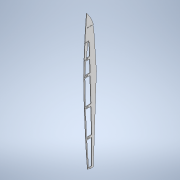
# Autodesk Inventor part: stinger
Saved by Autodesk Inventor 2020.3 (Build 243373010, 373A)
## iProperties
Created: 2020-05-20
Part Number: stinger
Material: Generic
Document SubType Name: Modeling
Designer: kardo
Density: 1 g/cm^3
Appearance: Default
Mass: 15.45 g
Surface Area: 197.993 cm^2
Volume: 15.45 cm^3
Author: kardo
Autodesk Inventor part; units mm, degrees
ref_plane "YZ Plane" through (0, 0, 0) normal (1, 0, 0) x (0, 1, 0)
ref_plane "XZ Plane" through (0, 0, 0) normal (0, 1, 0) x (-1, 0, 0)
ref_plane "XY Plane" through (0, 0, 0) normal (0, 0, 1) x (1, 0, 0)
derived "base_sketch.ipt"
sketch "stringer" plane through (0, 0, 0) normal (1, 0, 0) x (0, 1, 0)
  line L0 (-306, 11.475) -> (0, 0)
  line L1 (-306, 31.875) -> (-306, 11.475)
  line L2 (-412.4622, 0) -> (310.4457, 0)
  line L3 (0, -13.6228) -> (0, 64.3297)
  line L4 (0, 0) -> (122.4, 8.559)
  line L5 (-306, 31.875) -> (-153, 45.9) construction
  line L6 (-153, 45.9) -> (0, 45.9) construction
  line L7 (0, 45.9) -> (102, 45.9) construction
  line L8 (102, 45.9) -> (204, 35.7) construction
  line L9 (122.4, 8.559) -> (204, 14.2651) construction
  spline S0 degree 4 poles (-306, 31.875) (-229.6805, 38.871) (-153.0004, 41.6957) (-76.5755, 45.9) (0, 45.9) knots 0 0 0 0 0 1 1 1 1 1
  spline S1 degree 4 poles (0, 45.9) (51.0599, 45.9) (102.0004, 42.8427) (153.143, 40.7857) (204, 35.7) knots 0 0 0 0 0 1 1 1 1 1
  spline S2 degree 4 poles (122.4, 8.559) (129.6243, 9.0642) (155.3021, 10.8598) (183.5774, 20.1745) (192.0601, 27.4338) (204, 35.7) knots 0 0 0 0 0 0.281346 1 1 1 1 1
  point P0 (-153, 41.6925)
  point P1 (102, 42.84)
  point P2 (163.2, 15.056)
  point P3 (187.68, 24.9131)
sketch "bulkhead_main" plane through (0, 0, 0) normal (0, 1, 0) x (-1, 0, 0)
  line L0 (0, 19.935) -> (28.764, 19.935)
  line L1 (28.764, 19.935) -> (28.764, 13.529)
  line L2 (28.764, 13.529) -> (62.322, 13.529)
  line L3 (0, 0) -> (-11.5056, 0)
  line L4 (-11.5056, 0) -> (-11.5056, -2.4868)
  line L5 (-11.5056, -2.4868) -> (-34.5168, -2.4868)
  line L6 (-34.5168, -2.4868) -> (-57.528, 27.54)
  line L7 (19.176, 46.818) -> (62.322, 46.818)
  line L8 (0, 19.935) -> (0, 0)
  line L9 (86.7165, 0) -> (-84.045, 0)
  line L10 (0, -13.6228) -> (0, 64.3297)
  line L11 (62.322, 46.818) -> (62.322, 13.529)
  spline S0 degree 4 poles (-57.528, 27.54) (-46.0483, 34.2051) (-30.6129, 40.5281) (-11.2214, 45.0414) (8.3201, 46.818) (15.5662, 46.818) (19.176, 46.818) knots 0 0 0 0 0 0.630279 0.815816 1 1 1 1 1
  line L12 (0, 35.7) -> (-57.528, 27.54) construction
  line L13 (-11.5056, -2.4868) -> (0, -2.4868) construction
  line L14 (0, -2.4868) -> (0, 0) construction
  point P0 (0, 45.9)
  point P1 (-38.352, 36.72)
  point P2 (-19.176, 42.5952)
  point P3 (0, 13.529)
sketch "bulkhead_F1" plane through (0, 56.1, 0) normal (0, 1, 0) x (-1, 0, 0)
  line L0 (19.176, 46.818) -> (62.322, 46.818)
  line L1 (-34.5168, -2.4868) -> (-57.528, 27.54)
  line L2 (-11.5056, -2.4868) -> (-34.5168, -2.4868)
  line L3 (-11.5056, 0) -> (-11.5056, -2.4868)
  line L4 (0, 0) -> (-11.5056, 0)
  line L5 (62.322, 46.818) -> (62.322, 13.529)
  line L6 (28.764, 19.935) -> (28.764, 13.529)
  line L7 (-37.5231, 1.4361) -> (-11.5056, 1.4361)
  line L8 (-11.5056, 1.4361) -> (-11.5056, 3.9229)
  line L9 (-11.5056, 3.9229) -> (0, 3.9229)
  line L10 (0, 3.9229) -> (0, 21.6458)
  line L11 (0, 21.6458) -> (28.764, 21.6458)
  line L12 (28.764, 21.6458) -> (28.764, 14.7544)
  line L13 (28.764, 14.7544) -> (62.322, 14.7544)
  line L14 (62.322, 43.2359) -> (19.176, 43.2359)
  line L15 (-57.528, 27.54) -> (-37.5231, 1.4361)
  line L16 (0, 45.9) -> (0, 44.8052) construction
  line L17 (-19.176, 42.5952) -> (-19.176, 41.8654) construction
  line L18 (-38.352, 36.72) -> (-38.352, 36.3551) construction
  line L19 (0, 19.935) -> (0, 0)
  line L20 (0, 44.8052) -> (0, 42.3179)
  spline S0 degree 4 poles (-57.528, 27.54) (-46.0483, 34.2051) (-30.6129, 40.5281) (-11.2214, 45.0414) (8.3201, 46.818) (15.5662, 46.818) (19.176, 46.818) knots 0 0 0 0 0 0.630279 0.815816 1 1 1 1 1
  spline S1 degree 3 poles (-57.528, 27.54) (-39.1506, 37.8756) (-19.5945, 42.9173) (0, 44.8052) knots 0 0 0 0 1 1 1 1
  spline S2 degree 2 poles (0, 42.3179) (9.5715, 43.2359) (19.176, 43.2359) knots 0 0 0 1 1 1
  line L21 (0, 35.7) -> (-57.528, 27.54) construction
  line L22 (-11.5056, 1.4361) -> (0, 1.4361) construction
  line L23 (0, 1.4361) -> (0, 3.9229) construction
  point P0 (0, 14.7544)
sketch "bulkhead_front" plane through (0, 112.2, 33.6972) normal (0, 1, 0) x (-1, 0, 0)
  line L0 (-40.5295, -28.3381) -> (-11.5056, -28.3381)
  line L1 (-11.5056, -28.3381) -> (-11.5056, -25.8514)
  line L2 (-11.5056, -25.8514) -> (0, -25.8514)
  line L3 (19.176, 13.1208) -> (62.322, 13.1208)
  line L4 (-11.5056, -36.1839) -> (-34.5168, -36.1839)
  line L5 (-11.5056, -33.6972) -> (-11.5056, -36.1839)
  line L6 (0, -33.6972) -> (-11.5056, -33.6972)
  line L7 (-34.5168, -36.1839) -> (-57.528, -6.1572)
  line L8 (0, -13.7621) -> (28.764, -13.7621)
  line L9 (28.764, -20.1682) -> (62.322, -20.1682)
  line L10 (28.764, -13.7621) -> (28.764, -20.1682)
  line L11 (62.322, 13.1208) -> (62.322, -20.1682)
  line L12 (0, -13.7621) -> (0, -33.6972)
  line L13 (0, -25.8514) -> (0, -10.3406)
  line L14 (0, -10.3406) -> (62.322, -10.3406)
  line L15 (19.176, 0.918) -> (62.322, 0.918)
  line L16 (-38.352, 1.8276) -> (-38.352, 3.0228) construction
  line L17 (-19.176, 6.5076) -> (-19.176, 8.898) construction
  line L18 (0, 8.6171) -> (0, 12.2028) construction
  line L19 (-40.5295, -28.3381) -> (-57.528, -6.1572)
  line L20 (0, 8.6171) -> (0, 0)
  spline S0 degree 4 poles (-57.528, -6.1572) (-46.0483, 0.508) (-30.6129, 6.8309) (-11.2214, 11.3442) (8.3201, 13.1208) (15.5662, 13.1208) (19.176, 13.1208) knots 0 0 0 0 0 0.630279 0.815816 1 1 1 1 1
  spline S1 degree 3 poles (-57.528, -6.1572) (-39.0789, 3.4175) (-19.5173, 7.5799) (0, 8.6171) knots 0 0 0 0 1 1 1 1
  spline S2 degree 3 poles (0, 0) (6.37, 0.918) (12.773, 0.918) (19.176, 0.918) knots 0 0 0 0 1 1 1 1
  line L21 (0, 2.0028) -> (-57.528, -6.1572) construction
  line L22 (-11.5056, -28.3381) -> (0, -28.3381) construction
  line L23 (0, -28.3381) -> (0, -25.8514) construction
sketch "bulkhead_F2" plane through (0, 158.1, 33.6972) normal (0, 1, 0) x (-1, 0, 0)
  line L0 (19.176, 13.1208) -> (62.322, 13.1208)
  line L1 (62.322, 13.1208) -> (62.322, -20.1682)
  line L2 (0, -33.6972) -> (-11.5056, -33.6972)
  line L3 (-11.5056, -36.1839) -> (-34.5168, -36.1839)
  line L4 (-11.5056, -33.6972) -> (-11.5056, -36.1839)
  line L5 (-34.5168, -36.1839) -> (-57.528, -6.1572)
  line L6 (0, 5.8272) -> (0, -20.0113)
  line L7 (0, -20.0113) -> (-11.5056, -20.0113)
  line L8 (-11.5056, -20.0113) -> (-11.5056, -21.8764)
  line L9 (-11.5056, -21.8764) -> (-35.9142, -21.8764)
  line L10 (-35.9142, -21.8764) -> (-48.8988, -4.9332)
  line L11 (-57.528, -8.9984) -> (-57.528, -6.1572) construction
  line L12 (-38.352, 3.0228) -> (-38.352, -0.9966) construction
  line L13 (-19.176, 8.898) -> (-19.176, 3.7072) construction
  line L14 (0, 12.2028) -> (0, 5.8272) construction
  spline S0 degree 4 poles (-57.528, -6.1572) (-46.0483, 0.508) (-30.6129, 6.8309) (-11.2214, 11.3442) (8.3201, 13.1208) (15.5662, 13.1208) (19.176, 13.1208) knots 0 0 0 0 0 0.630279 0.815816 1 1 1 1 1
  spline S1 degree 3 poles (-57.528, -8.9984) (-39.0792, 0.5819) (-19.5206, 4.7923) (0, 5.8272) knots 0 0 0 0 1 1 1 1
  line L15 (0, 2.0028) -> (-57.528, -6.1572) construction
  line L16 (0, 19.4965) -> (0, 13.1208) construction
  line L17 (0, 13.1208) -> (-57.528, 13.1208) construction
  line L18 (-57.528, 13.1208) -> (-57.528, 15.9621) construction
  line L19 (-57.528, 15.9621) -> (0, 19.4965) construction
  line L20 (-38.352, 17.1402) -> (-38.352, 13.1208) construction
  line L21 (-19.176, 18.3184) -> (-19.176, 13.1208) construction
  line L22 (-48.8988, -4.9332) -> (-48.8988, -1.5617) construction
  line L23 (-48.8988, 16.4923) -> (-48.8988, 13.1208) construction
  line L24 (-11.5056, -21.8764) -> (0, -21.8764) construction
  line L25 (0, -21.8764) -> (0, -20.0113) construction
sketch "bulkhead_B1" plane through (0, -102, 0) normal (0, 1, 0) x (-1, 0, 0)
  line L0 (19.176, 46.818) -> (62.322, 46.818)
  line L1 (0, 19.935) -> (0, 0)
  line L2 (62.322, 46.818) -> (62.322, 13.529)
  line L3 (0, 5.6919) -> (-27.3644, 38.3035)
  line L4 (62.322, 44.7066) -> (19.176, 44.7066)
  line L5 (-38.352, 36.72) -> (-38.352, 34.6086) construction
  line L6 (-19.176, 42.5952) -> (-19.176, 40.4838) construction
  line L7 (0, 45.9) -> (0, 43.7886) construction
  line L8 (19.176, 46.818) -> (19.176, 44.7066) construction
  line L9 (0, 19.935) -> (28.764, 19.935)
  line L10 (28.764, 19.935) -> (28.764, 13.529)
  line L11 (28.764, 13.529) -> (62.322, 13.529)
  line L12 (62.322, 13.7901) -> (28.764, 13.7901)
  line L13 (28.764, 13.7901) -> (28.764, 16.8245)
  line L14 (28.764, 16.8245) -> (0, 16.8245)
  line L15 (0, 16.8245) -> (0, 5.6919)
  spline S0 degree 4 poles (-57.528, 27.54) (-46.0483, 34.2051) (-30.6129, 40.5281) (-11.2214, 45.0414) (8.3201, 46.818) (15.5662, 46.818) (19.176, 46.818) knots 0 0 0 0 0 0.630279 0.815816 1 1 1 1 1
  spline S1 degree 3 poles (19.176, 44.7066) (-0.1981, 44.9447) (-19.6083, 41.6917) (-38.352, 34.6086) knots 0 0 0 0 1 1 1 1
  point P0 (0, 3.825)
  point P1 (0, 13.7901)
sketch "bulkhead_B2" plane through (0, -204, 0) normal (0, 1, 0) x (-1, 0, 0)
  line L0 (19.176, 46.818) -> (62.322, 46.818)
  line L1 (0, 19.935) -> (28.764, 19.935)
  line L2 (28.764, 13.529) -> (62.322, 13.529)
  line L3 (28.764, 19.935) -> (28.764, 13.529)
  line L4 (62.322, 46.818) -> (62.322, 13.529)
  line L5 (0, 9.5169) -> (0, 14.025)
  line L6 (0, 14.025) -> (62.322, 14.025)
  line L7 (0, 9.5169) -> (-21.5668, 35.2191)
  line L8 (62.322, 40.0294) -> (19.176, 40.0294)
  line L9 (-19.176, 35.8066) -> (-19.176, 42.5952) construction
  line L10 (-38.352, 36.72) -> (-38.352, 29.9314) construction
  line L11 (19.176, 46.818) -> (19.176, 40.0294) construction
  line L12 (0, 45.9) -> (0, 39.1114) construction
  spline S0 degree 4 poles (-57.528, 27.54) (-46.0483, 34.2051) (-30.6129, 40.5281) (-11.2214, 45.0414) (8.3201, 46.818) (15.5662, 46.818) (19.176, 46.818) knots 0 0 0 0 0 0.630279 0.815816 1 1 1 1 1
  spline S1 degree 3 poles (19.176, 40.0294) (-0.1981, 40.2675) (-19.6083, 37.0145) (-38.352, 29.9314) knots 0 0 0 0 1 1 1 1
  point P0 (0, 0)
  point P1 (0, 7.65)
  point P2 (0, 7.65)
sketch "transom" plane through (0, -306, 31.875) normal (0, 1, 0) x (-1, 0, 0)
  line L0 (19.176, 14.943) -> (62.322, 14.943)
  line L1 (62.322, 14.943) -> (62.322, -18.346)
  line L2 (28.764, -18.346) -> (62.322, -18.346)
  line L3 (0, -18.5331) -> (-13.7701, -2.1226)
  line L4 (0, -18.5331) -> (0, -17.85)
  line L5 (0, -17.85) -> (62.322, -17.85)
  line L6 (62.322, 0.918) -> (19.176, 0.918)
  line L7 (19.176, 14.943) -> (19.176, 0.918) construction
  line L8 (-19.176, -3.3048) -> (-19.176, 10.7202) construction
  line L9 (-38.352, 4.845) -> (-38.352, -9.18) construction
  line L10 (0, 14.025) -> (0, 0) construction
  spline S0 degree 4 poles (-57.528, -4.335) (-46.0483, 2.3301) (-30.6129, 8.6531) (-11.2214, 13.1664) (8.3201, 14.943) (15.5662, 14.943) (19.176, 14.943) knots 0 0 0 0 0 0.630279 0.815816 1 1 1 1 1
  spline S1 degree 3 poles (19.176, 0.918) (-0.1981, 1.1561) (-19.6083, -2.0969) (-38.352, -9.18) knots 0 0 0 0 1 1 1 1
  line L11 (0, 0) -> (0, -20.4)
  point P0 (0, -31.875)
sketch "stringer_inside" plane through (0, 0, 0) normal (1, 0, 0) x (0, 1, 0)
  line L0 (-306, 31.875) -> (-306, 11.475)
  line L1 (0, 0) -> (122.4, 8.559)
  line L2 (-306, 14.025) -> (-193.8, 14.025)
  line L3 (112.2, 23.3566) -> (112.2, 33.6972)
  line L4 (0, 45.9) -> (56.7636, 45.9) construction
  line L5 (56.7636, 45.9) -> (112.2, 33.6972) construction
  line L6 (112.2, 42.3143) -> (112.2, 7.8458) construction
  line L7 (0, -13.6228) -> (0, 64.3297)
  line L8 (-193.8, 14.025) -> (112.2, 23.3566)
  line L9 (-193.8, 14.025) -> (0, 13.529)
  line L10 (17.2125, 13.5685) -> (112.2, 16.4652)
  line L11 (0, 13.529) -> (-0.1952, 19.9291) construction
  line L12 (17.2125, 13.5685) -> (17.0025, 20.4535) construction
  spline S0 degree 4 poles (0, 45.9) (51.0599, 45.9) (102.0004, 42.8427) (153.143, 40.7857) (204, 35.7) knots 0 0 0 0 0 1 1 1 1 1
  spline S1 degree 3 poles (0, 45.9) (37.8279, 45.9) (75.6167, 40.2679) (112.2, 33.6972) knots 0 0 0 0 1 1 1 1
  spline S2 degree 4 poles (0, 13.529) (2.1516, 13.5235) (6.4547, 13.5125) (10.7595, 13.3717) (15.0615, 13.5029) (17.2125, 13.5685) knots 0 0 0 0 0 0.5 1 1 1 1 1
  point P0 (56.7636, 42.2391)
sketch "stinger_bottom_liner" plane through (0, 0, 0) normal (1, 0, 0) x (0, 1, 0)
  line L0 (0, -2.4868) -> (56.1, 1.4361)
  line L1 (56.1, 1.4361) -> (112.2, 5.359)
  line L2 (112.2, 5.359) -> (122.4, 6.0723)
  line L3 (0, -2.4868) -> (0, 0) construction
  line L4 (56.1, 1.4361) -> (56.1, 3.9229) construction
  line L5 (112.2, 5.359) -> (112.2, 7.8458) construction
  line L6 (158.1, 11.8207) -> (158.1, 13.6858) construction
  line L7 (0, 0) -> (122.4, 8.559)
  spline S0 degree 4 poles (122.4, 6.0723) (129.6678, 6.5805) (155.5572, 8.3909) (183.6316, 19.8242) (192.0814, 26.863) (204, 35.7) knots 0 0 0 0 0 0.280728 1 1 1 1 1
  spline S1 degree 4 poles (122.4, 8.559) (129.6243, 9.0642) (155.3021, 10.8598) (183.5774, 20.1745) (192.0601, 27.4338) (204, 35.7) knots 0 0 0 0 0 0.281346 1 1 1 1 1
  point P0 (163.2, 13.3976)
  point P1 (187.68, 24.2914)
  point P2 (187.68, 24.9131)
  point P3 (163.2, 15.056)
sketch "Sketch9" plane through (0, 0, 0) normal (1, 0, 0) x (0, 1, 0)
  spline S0 degree 4 poles (-306, 31.875) (-229.6805, 38.871) (-153.0004, 41.6957) (-76.5755, 45.9) (0, 45.9) knots 0 0 0 0 0 1 1 1 1 1 projected
  line L0 (-306, 11.475) -> (0, 0) projected
  line L1 (0, 0) -> (122.4, 8.559) projected
  spline S1 degree 4 poles (122.4, 8.559) (129.6243, 9.0642) (155.3021, 10.8598) (183.5774, 20.1745) (192.0601, 27.4338) (204, 35.7) knots 0 0 0 0 0 0.281346 1 1 1 1 1 projected
  spline S2 degree 4 poles (0, 45.9) (51.0599, 45.9) (102.0004, 42.8427) (153.143, 40.7857) (204, 35.7) knots 0 0 0 0 0 1 1 1 1 1 projected
  line L2 (158.1, 39.5244) -> (158.1, 13.6858) projected
  line L3 (-306, 11.475) -> (-306, 14.025) projected
  line L4 (-306, 14.025) -> (-306, 23.0411)
  line L5 (-306, 23.0411) -> (-304, 23.0411)
  line L6 (-304, 23.0411) -> (-304, 32.0573)
  line L7 (0, 19.935) -> (0, 0) projected
  line L8 (0, 45.9) -> (0, 32.9175)
  line L9 (0, 32.9175) -> (2, 32.9175)
  line L10 (2, 32.9175) -> (2, 45.8983)
  line L11 (0, 32.9175) -> (0, 19.935) construction
  line L12 (-204, 7.65) -> (-204, 14.025) projected
  line L13 (56.1, 3.9229) -> (56.1, 21.6458) projected
  line L14 (112.2, 7.8458) -> (112.2, 23.3566) projected
  line L15 (-102, 16.8245) -> (-102, 3.825) projected
  line L16 (-102, 16.8245) -> (-102, 30.3066) construction
  line L17 (-102, 30.3066) -> (-102, 43.7886)
  line L18 (-102, 30.3066) -> (-100, 30.3066)
  line L19 (-100, 30.3066) -> (-100, 43.8602)
  line L20 (-204, 14.025) -> (-204, 26.5682) construction
  line L21 (-204, 26.5682) -> (-204, 39.1114)
  line L22 (-204, 26.5682) -> (-202, 26.5682)
  line L23 (-202, 26.5682) -> (-202, 39.2223)
  line L24 (56.1, 21.6458) -> (56.1, 31.9819) construction
  line L25 (56.1, 31.9819) -> (56.1, 42.3179)
  line L26 (56.1, 31.9819) -> (54.1, 31.9819)
  line L27 (54.1, 31.9819) -> (54.1, 44.8737)
  line L28 (112.2, 23.3566) -> (112.2, 28.5269) construction
  line L29 (112.2, 28.5269) -> (112.2, 33.6972)
  line L30 (156.1, 34.3566) -> (158.1, 34.3566)
  line L31 (158.1, 34.3566) -> (158.1, 29.1889)
  line L32 (158.1, 29.1889) -> (156.1, 29.1889)
  line L33 (156.1, 24.0212) -> (158.1, 24.0212)
  line L34 (158.1, 24.0212) -> (158.1, 18.8535)
  line L35 (158.1, 18.8535) -> (156.1, 18.8535)
  line L36 (156.1, 29.1889) -> (156.1, 34.3566)
  line L37 (156.1, 24.0212) -> (156.1, 18.8535)
  line L38 (158.1, 34.3566) -> (158.1, 39.5244) construction
  line L39 (158.1, 29.1889) -> (158.1, 24.0212) construction
  line L40 (158.1, 18.8535) -> (158.1, 13.6858) construction
  line L41 (-306, 31.875) -> (-204, 39.1114) construction
  line L42 (-301, 27.359) -> (-301, 19.025)
  line L43 (-299, 17.025) -> (-209, 17.025)
  line L44 (-207, 19.025) -> (-207, 33.7441)
  line L45 (-209.1415, 35.7391) -> (-299.1415, 29.354)
  line L46 (-199, 34.4454) -> (-199, 18.9297)
  line L47 (-196.939, 16.9307) -> (-106.939, 19.6753)
  line L48 (-105, 21.6743) -> (-105, 38.5551)
  line L49 (-107.0912, 40.553) -> (-197.0912, 36.4434)
  line L50 (-97, 38.9611) -> (-97, 22.0403)
  line L51 (-3, 24.7849) -> (-3, 40.797)
  line L52 (-5.0408, 42.7966) -> (-95.0408, 40.9607)
  line L53 (-202, 39.2223) -> (-102, 43.7886) construction
  line L54 (-100, 43.8602) -> (0, 45.9) construction
  arc A0 (-301, 19.025) -> (-299, 17.025) centre (-299, 19.025) ccw
  arc A1 (-299.1415, 29.354) -> (-301, 27.359) centre (-299, 27.359) ccw
  arc A2 (-207, 33.7441) -> (-209.1415, 35.7391) centre (-209, 33.7441) ccw
  arc A3 (-209, 17.025) -> (-207, 19.025) centre (-209, 19.025) ccw
  arc A4 (-199, 18.9297) -> (-196.939, 16.9307) centre (-197, 18.9297) ccw
  arc A5 (-197.0912, 36.4434) -> (-199, 34.4454) centre (-197, 34.4454) ccw
  arc A6 (-105, 38.5551) -> (-107.0912, 40.553) centre (-107, 38.5551) ccw
  arc A7 (-106.939, 19.6753) -> (-105, 21.6743) centre (-107, 21.6743) ccw
  arc A8 (-97, 22.0403) -> (-94.939, 20.0412) centre (-95, 22.0403) ccw
  arc A9 (-95.0408, 40.9607) -> (-97, 38.9611) centre (-95, 38.9611) ccw
  arc A10 (-3, 40.797) -> (-5.0408, 42.7966) centre (-5, 40.797) ccw
  arc A11 (-4.939, 22.7858) -> (-3, 24.7849) centre (-5, 24.7849) ccw
  line L55 (-193.8, 14.025) -> (112.2, 23.3566) projected
  spline S3 degree 3 poles (0, 45.9) (37.8279, 45.9) (75.6167, 40.2679) (112.2, 33.6972) knots 0 0 0 0 1 1 1 1 projected
  line L56 (0, 45.9) -> (56.7636, 42.2391) construction
  line L57 (56.7636, 42.2391) -> (112.2, 33.6972) construction
  line L58 (5, 40.4382) -> (5, 25.1508)
  line L59 (7.061, 23.1517) -> (49.161, 24.4356)
  line L60 (51.1, 26.4347) -> (51.1, 37.723)
  line L61 (49.2287, 39.7189) -> (7.1287, 42.434)
  line L62 (59.1, 36.512) -> (59.1, 26.8006)
  line L63 (61.161, 24.8016) -> (105.261, 26.1464)
  line L64 (107.2, 28.1455) -> (107.2, 29.7168)
  line L65 (105.5046, 31.6934) -> (61.4046, 38.4886)
  arc A12 (49.161, 24.4356) -> (51.1, 26.4347) centre (49.1, 26.4347) ccw
  arc A13 (5, 25.1508) -> (7.061, 23.1517) centre (7, 25.1508) ccw
  arc A14 (7.1287, 42.434) -> (5, 40.4382) centre (7, 40.4382) ccw
  arc A15 (51.1, 37.723) -> (49.2287, 39.7189) centre (49.1, 37.723) ccw
  arc A16 (61.4046, 38.4886) -> (59.1, 36.512) centre (61.1, 36.512) ccw
  arc A17 (59.1, 26.8006) -> (61.161, 24.8016) centre (61.1, 26.8006) ccw
  arc A18 (105.261, 26.1464) -> (107.2, 28.1455) centre (105.2, 28.1455) ccw
  arc A19 (107.2, 29.7168) -> (105.5046, 31.6934) centre (105.2, 29.7168) ccw
  line L66 (112.2, 33.6972) -> (112.2, 42.3143)
  line L67 (56.1, 42.3179) -> (56.1, 44.8052)
  line L68 (112.2, 28.5269) -> (110.2, 28.5269)
  line L69 (110.2, 28.5269) -> (110.2, 42.4198)
  spline S4 degree 4 poles (122.4, 6.0723) (129.6678, 6.5805) (155.5572, 8.3909) (183.6316, 19.8242) (192.0814, 26.863) (204, 35.7) knots 0 0 0 0 0 0.280728 1 1 1 1 1 projected
  line L70 (156.1, 13.1963) -> (156.1, 11.2554)
  line L71 (-306, 14.025) -> (-193.8, 14.025) projected
  line L72 (-94.939, 20.0412) -> (-4.939, 22.7858)
  point P0 (2, 45.8948)
  point P1 (54.1, 42.551)
  point P2 (158.1, 18.8535)
  dimension "d1" = 2
  dimension "d2" = 2
  dimension "d5" = 2
  dimension "d6" = 2
  dimension "d9" = 2
  dimension "d10" = 2
  dimension "d25" = 3
  dimension "d26" = 3
  dimension "d27" = 3
  dimension "d28" = 3
  dimension "d30" = 3
  dimension "d31" = 3
  dimension "d32" = 3
  dimension "d33" = 3
  dimension "d35" = 3
  dimension "d36" = 2
  dimension "d37" = 3
  dimension "d38" = 3
  dimension "d39" = 3
  dimension "d40" = 3
  dimension "d43" = 3
  dimension "d45" = 2
  dimension "d46" = 2
  dimension "d47" = 3
  dimension "d48" = 2
  dimension "d49" = 3
  dimension "d50" = 3
  dimension "d52" = 3
  dimension "d53" = 3
  dimension "d54" = 3
  constraints: 124 end point, 40 point on circle, 40 tangent, 21 parallel, 20 centre point, 18 equal radius, 18 vertical, 10 equal length, 9 horizontal, 5 point on line, 2 collinear, 2 perpendicular, 15 other
  measures "d1" distance of L4.end L5.end
  measures "d2" distance of L8.end L9.end
  measures "d5" distance of L20.end L22.end
  measures "d6" distance of L16.end L18.end
  measures "d9" distance of L33.start L33.end
  measures "d10" distance of L31.end L32.end
  measures "d25" distance between parallel lines of L6 L42
  measures "d26" distance between parallel lines of L41 L45
  measures "d27" distance between parallel lines of L20 L44
  measures "d28" distance between parallel lines of L46 L23
  measures "d30" distance between parallel lines of L53 L49
  measures "d31" distance between parallel lines of L16 L48
  measures "d32" distance between parallel lines of L19 L50
  measures "d33" distance between parallel lines of L54 L52
  measures "d35" distance between parallel lines of L11 L51
  measures "d36" radius of A0
  measures "d37" distance between parallel lines of L55 L63
  measures "d38" distance between parallel lines of L55 L59
  measures "d39" distance between parallel lines of L10 L58
  measures "d40" distance between parallel lines of L56 L61
  measures "d43" distance between parallel lines of L57 L65
  measures "d45" radius of A12
  measures "d46" distance of L28.end L68.end
  measures "d47" distance between parallel lines of L69 L64
  measures "d48" distance of L24.end L26.end
  measures "d49" distance between parallel lines of L27 L60
  measures "d50" distance between parallel lines of L62 L25
  measures "d52" distance between parallel lines of L43 L71
  measures "d53" distance between parallel lines of L55 L47
  measures "d54" distance between parallel lines of L55 L72
extrude "Extrusion1" add sketch "Sketch9" against normal blind 2 contours S0 L21 L22 L23 L17 L18 L19 L8 L9 L10 S3 L27 L26 L25 L69 L68 L29 L66 S2 L2 L30 L36 L32 L33 L37 L35 S1 L1 L14 L55 L71 L4 L5 L6 | L71 L12 L0 L3 | L71 L55 L15 L0 L12 | S2 L27 S3 L10 | L15 L55 L7 L0 | L7 L55 L13 L1 | S2 L69 S3 L67 | L13 L55 L14 L1 | S2 S1 L2 | S1 S4 L70
equation "\"d1\" = bulkhead_thickness"
equation "\"d2\" = bulkhead_thickness"
equation "\"d5\" = bulkhead_thickness"
equation "\"d6\" = bulkhead_thickness"
equation "\"d9\" = bulkhead_thickness"
equation "\"d10\" = bulkhead_thickness"
equation "\"d46\" = bulkhead_thickness"
equation "\"d48\" = bulkhead_thickness"
equation "\"bulkhead_thickness\" = 2"
body "Solid1"
